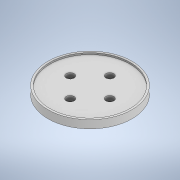
# Autodesk Inventor part: GNSS_mount
Saved by Autodesk Inventor 2021.4 (Build 254397000, 397)
## iProperties
Created: 2023-11-07
Part Number: GNSS_mount
Material: 一般
Document SubType Name: Modeling
Designer: ryusei
Density: 1 g/cm^3
Appearance: 既定
Author: ryusei
Autodesk Inventor part; units mm, degrees
ref_plane "YZ Plane" through (0, 0, 0) normal (1, 0, 0) x (0, 1, 0)
ref_plane "XZ Plane" through (0, 0, 0) normal (0, 1, 0) x (-1, 0, 0)
ref_plane "XY Plane" through (0, 0, 0) normal (0, 0, 1) x (1, 0, 0)
sketch "スケッチ1" plane through (0, 0, 0) normal (0, 1, 0) x (-1, 0, 0)
  circle A0 centre (0, 0) radius 53
  dimension "d0" = 106
  constraints: 1 centre point, 1 coincident
  measures "d0" diameter of A0
extrude "押し出し1" add sketch "スケッチ1" along normal blind 10
sketch "スケッチ2" plane through (0, 10, 0) normal (0, 1, 0) x (1, 0, 0)
  circle A0 centre (0, 0) radius 50.5
  dimension "d3" = 101
  constraints: 1 centre point, 1 coincident
  measures "d3" diameter of A0
extrude "押し出し2" cut sketch "スケッチ2" against normal blind 2
sketch "スケッチ3" plane through (0, 8, 0) normal (0, 1, 0) x (1, 0, 0)
  point P0 (0, 0)
  point P1 (25, 0)
  point P2 (0, 25)
  point P3 (-25, 0)
  point P4 (0, -25)
  dimension "d6" = 25
  dimension "d9" = 360
  constraints: 5 other
  measures "d6" distance of point (25, 0) point (0, 0)
hole "穴1" at (25, 8, 0) at (0, 8, -25) at (-25, 8, 0) at (0, 8, 25) direction (0, -1, 0) diameter 6 end through all
hole "穴2" at (-25, 8, 0) at (0, 8, -25) at (25, 8, 0) at (0, 8, 25) direction (0, -1, 0) diameter 6 end through all counterbore diameter 10 counterbore depth 5
